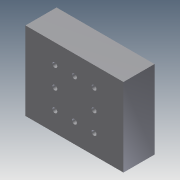
# Autodesk Inventor part: hconnector
Saved by Autodesk Inventor 2011 (Build 150239000, 239)
## iProperties
Created: 2011-12-11
Part Number: hconnector
Document SubType Name: Modeling
Designer: Matthew
Density: 1 g/cm^3
Author: Matthew
Autodesk Inventor part; units mm, degrees
ref_plane "YZ Plane" through (0, 0, 0) normal (1, 0, 0) x (0, 1, 0)
ref_plane "XZ Plane" through (0, 0, 0) normal (0, 1, 0) x (-1, 0, 0)
ref_plane "XY Plane" through (0, 0, 0) normal (0, 0, 1) x (1, 0, 0)
sketch "Sketch1" plane through (0, 0, 0) normal (0, 0, 1) x (1, 0, 0)
  line L0 (-15.9035, 8.2993) -> (24.0965, 8.2993)
  line L1 (24.0965, 8.2993) -> (24.0965, -21.7007)
  line L2 (24.0965, -21.7007) -> (-15.9035, -21.7007)
  line L3 (-15.9035, -21.7007) -> (-15.9035, 8.2993)
  point P0 (0, 0)
  dimension "d0" = 40
  dimension "d1" = 30
  constraints: 8 end point, 2 parallel, 1 horizontal, 1 perpendicular
  measures "d0" distance of L1.end L2.end
  measures "d1" distance of L0.end L1.end
extrude "Extrusion1" add sketch "Sketch1" along normal blind 2
sketch "Sketch2" plane through (0, 0, 2) normal (0, 0, 1) x (1, 0, 0)
  line L0 (-15.9035, -21.7007) -> (-15.9035, 8.2993) projected
  line L1 (24.0965, -21.7007) -> (-15.9035, -21.7007) projected
  line L2 (-15.9035, -6.7007) -> (4.0965, -6.7007)
  line L3 (4.0965, -6.7007) -> (4.0965, -14.7007)
  line L4 (4.0965, -14.7007) -> (-3.9035, -14.7007)
  line L5 (-3.9035, -14.7007) -> (-3.9035, 1.2993)
  line L6 (-3.9035, 1.2993) -> (12.0965, 1.2993)
  line L7 (12.0965, 1.2993) -> (12.0965, -14.7007)
  circle A0 centre (12.0965, -6.7007) radius 1
  circle A1 centre (12.0965, 1.2993) radius 1
  circle A2 centre (4.0965, 1.2993) radius 1
  circle A3 centre (-3.9035, 1.2993) radius 1
  circle A4 centre (-3.9035, -6.7007) radius 1
  circle A5 centre (-3.9035, -14.7007) radius 1
  circle A6 centre (4.0965, -14.7007) radius 1
  circle A7 centre (12.0965, -14.7007) radius 1
  point P0 (0, 0)
  dimension "d4" = 8
  dimension "d5" = 8
  dimension "d6" = 16
  dimension "d7" = 16
  dimension "d8" = 16
  dimension "d9" = 2
  constraints: 12 end point, 8 centre point, 5 coincident, 5 parallel, 4 midpoint, 1 perpendicular
  measures "d4" distance of L2.end L3.end
  measures "d5" distance of L3.end L4.end
  measures "d6" distance of L4.end L5.end
  measures "d7" distance of L5.end L6.end
  measures "d8" distance of L6.end L7.end
  measures "d9" diameter of A0
extrude "Extrusion2" cut sketch "Sketch2" against normal blind 2 contours A7 | A0 L7 | L7 A0 | A1 L7 L6 | L6 L7 A1 | A2 L6 | L6 A2 | A3 L6 L5 | L5 L6 A3 | A4 L5 L2 | L2 L5 A4 | L5 A4 L2 | L2 A4 L5 | A6 L4 L3 | L3 L4 A6 | A5 L4 L5 | L5 L4 A5
sketch "Sketch3" plane through (-15.9035, -21.7007, 0) normal (0, -1, 0) x (1, 0, 0)
  line L0 (40, 2) -> (0, 2) projected
  line L1 (0, 0) -> (0, 2) projected
  line L2 (40, 0) -> (0, 0) projected
  line L3 (40, 0) -> (40, 2) projected
  point P0 (15.9035, 0)
extrude "Extrusion3" add sketch "Sketch3" along normal blind 1
sketch "Sketch4" plane through (-15.9035, 8.2993, 0) normal (0, 1, 0) x (1, 0, 0)
  line L0 (0, -2) -> (40, -2) projected
  line L1 (40, 0) -> (40, -2) projected
  line L2 (0, 0) -> (40, 0) projected
  line L3 (0, 0) -> (0, -2) projected
  point P0 (15.9035, 0)
extrude "Extrusion4" add sketch "Sketch4" along normal blind 1
sketch "Sketch5" plane through (0, 0, 2) normal (0, 0, 1) x (1, 0, 0)
  circle A0 centre (12.0965, -14.7007) radius 1 projected
  circle A1 centre (4.0965, -14.7007) radius 1 projected
  circle A2 centre (-3.9035, -14.7007) radius 1 projected
  circle A3 centre (-3.9035, -6.7007) radius 1 projected
  circle A4 centre (-3.9035, 1.2993) radius 1 projected
  circle A5 centre (4.0965, 1.2993) radius 1 projected
  circle A6 centre (12.0965, 1.2993) radius 1 projected
  circle A7 centre (12.0965, -6.7007) radius 1 projected
  line L0 (24.0965, 9.2993) -> (24.0965, -22.7007) projected
  line L1 (24.0965, 9.2993) -> (-15.9035, 9.2993) projected
  line L2 (-15.9035, -22.7007) -> (-15.9035, 9.2993) projected
  line L3 (-15.9035, -22.7007) -> (24.0965, -22.7007) projected
  point P0 (0, 0)
extrude "Extrusion5" add sketch "Sketch5" along normal blind 9.525
sketch "Sketch6" plane through (0, 0, 0) normal (0, 0, -1) x (-1, 0, 0)
  circle A0 centre (-12.0965, -14.7007) radius 1 projected
  circle A1 centre (-4.0965, -14.7007) radius 1 projected
  circle A2 centre (3.9035, -14.7007) radius 1 projected
  circle A3 centre (3.9035, -6.7007) radius 1 projected
  circle A4 centre (3.9035, 1.2993) radius 1 projected
  circle A5 centre (-4.0965, 1.2993) radius 1 projected
  circle A6 centre (-12.0965, 1.2993) radius 1 projected
  circle A7 centre (-12.0965, -6.7007) radius 1 projected
  line L0 (-24.0965, 9.2993) -> (-24.0965, -22.7007) projected
  line L1 (-24.0965, -22.7007) -> (15.9035, -22.7007) projected
  line L2 (15.9035, -22.7007) -> (15.9035, 9.2993) projected
  line L3 (15.9035, 9.2993) -> (-24.0965, 9.2993) projected
  point P0 (0, 0)
extrude "Extrusion6" add sketch "Sketch6" along normal blind 1.1684
sketch "Sketch7" plane through (-15.9035, -22.7007, 0) normal (0, -1, 0) x (1, 0, 0)
  line L0 (40, 11.525) -> (0, 11.525) projected
  line L1 (0, -1.1684) -> (1, -1.1684)
  line L2 (1, -1.1684) -> (1, 11.525)
  line L3 (1, 11.525) -> (0, 11.525)
  line L4 (0, 11.525) -> (0, -1.1684)
  point P0 (15.9035, 0)
  dimension "d20" = 1
  constraints: 8 end point, 2 parallel, 1 horizontal, 1 perpendicular, 1 point on line
  measures "d20" distance of L3.end L2.end
extrude "Extrusion7" cut sketch "Sketch7" against normal blind 50.8
body "Solid1"
